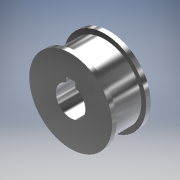
# Autodesk Inventor part: HTD5M 25 Pulley
Saved by Autodesk Inventor 2019.4 (Build 234330000, 330)
## iProperties
Created: 2019-12-31
Part Number: HTD5M 25 Pulley
Material: Aluminum 6061
Document SubType Name: Modeling
Designer: Mark
Mass: 63.0993 g
Surface Area: 73.2246 cm^2
Volume: 23.3701 cm^3
Density: 2.7 g/cm^3
Appearance: Aluminum - Flat
Author: Mark
Autodesk Inventor part; units mm, degrees
ref_plane "YZ Plane" through (0, 0, 0) normal (1, 0, 0) x (0, 1, 0)
ref_plane "XZ Plane" through (0, 0, 0) normal (0, 1, 0) x (-1, 0, 0)
ref_plane "XY Plane" through (0, 0, 0) normal (0, 0, 1) x (1, 0, 0)
sketch "Sketch1" plane through (0, 0, 0) normal (0, 0, 1) x (1, 0, 0)
  circle A0 centre (0, 0) radius 22.5
  dimension "d0" = 45
  constraints: 1 centre point, 1 coincident
  measures "d0" diameter of A0
extrude "Extrusion1" add sketch "Sketch1" along normal blind 2.5
sketch "Sketch2" plane through (0, 0, 2.5) normal (0, 0, 1) x (1, 0, 0)
  circle A0 centre (0, 0) radius 19.895
  dimension "d3" = 39.79
  constraints: 1 centre point, 1 coincident
  measures "d3" diameter of A0
extrude "Extrusion2" add sketch "Sketch2" along normal blind 16
sketch "Sketch3" plane through (0, 0, 18.5) normal (0, 0, 1) x (1, 0, 0)
  circle A0 centre (0, 0) radius 22.5
  dimension "d6" = 45
  constraints: 1 centre point, 1 coincident
  measures "d6" diameter of A0
extrude "Extrusion3" add sketch "Sketch3" along normal blind 2.5
sketch "Sketch4" plane through (0, 0, 21) normal (0, 0, 1) x (1, 0, 0)
  circle A0 centre (0, 0) radius 8
  line L0 (-2.5, 5.7) -> (2.5, 5.7)
  line L1 (2.5, 5.7) -> (2.5, 10.3)
  line L2 (2.5, 10.3) -> (-2.5, 10.3)
  line L3 (-2.5, 10.3) -> (-2.5, 5.7)
  line L4 (-2.5, 5.7) -> (2.5, 10.3) construction
  line L5 (2.5, 5.7) -> (-2.5, 10.3) construction
  point P0 (0, 8)
  dimension "d9" = 16
  dimension "d10" = 5
  dimension "d11" = 4.6
  constraints: 12 end point, 2 midpoint, 2 parallel, 1 coincident, 1 horizontal, 1 perpendicular, 1 vertical alignment, 2 other
  measures "d10" distance of L2.end L1.end
  measures "d11" distance of L1.end L0.end
extrude "Extrusion4" cut sketch "Sketch4" against normal blind 21
body "Solid1"
